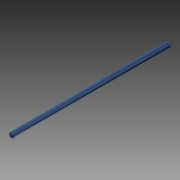
# Autodesk Inventor part: TUBO
Saved by Autodesk Inventor 2015 (Build 190159000, 159)
## iProperties
Created: 2016-03-04
Part Number: TUBO
Material: Generic
Document SubType Name: Modeling
Designer: Everton
Density: 1 g/cm^3
Appearance: Default
Author: Everton
Autodesk Inventor part; units mm, degrees
ref_plane "YZ Plane" through (0, 0, 0) normal (1, 0, 0) x (0, 1, 0)
ref_plane "XZ Plane" through (0, 0, 0) normal (0, 1, 0) x (-1, 0, 0)
ref_plane "XY Plane" through (0, 0, 0) normal (0, 0, 1) x (1, 0, 0)
sketch "Sketch1" plane through (0, 0, 0) normal (0, 1, 0) x (-1, 0, 0)
  circle A0 centre (0, 0) radius 29
  dimension "d0" = 58
  constraints: 1 centre point, 1 coincident
  measures "d0" diameter of A0
extrude "Extrusion1" add sketch "Sketch1" along normal blind 1800
fillet "Fillet1" radius 20 2 edges at (29, 1800, 0) (29, 0, 0)
body "Solid1"
